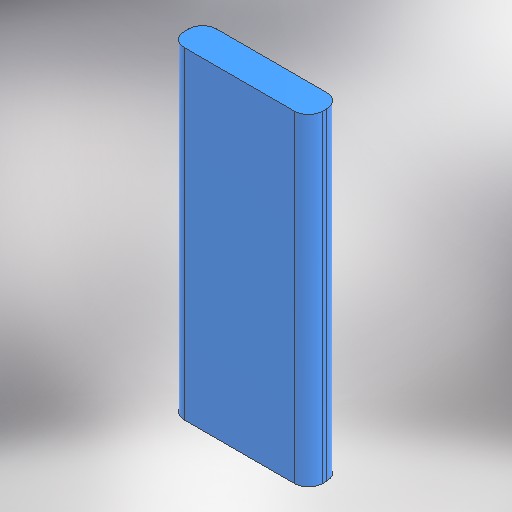
# Autodesk Inventor part: iPod Nano
Saved by Autodesk Inventor 2026.2 (Build 302298000, 298)
## iProperties
Created: 2026-01-13
Part Number: iPod Nano
Material: Generic
Document SubType Name: Modeling
Designer: andyeske
Density: 1 g/cm^3
Appearance: Default
Author: andyeske
Autodesk Inventor part; units mm, degrees
ref_plane "YZ Plane" through (0, 0, 0) normal (1, 0, 0) x (0, 1, 0)
ref_plane "XZ Plane" through (0, 0, 0) normal (0, 1, 0) x (-1, 0, 0)
ref_plane "XY Plane" through (0, 0, 0) normal (0, 0, 1) x (1, 0, 0)
sketch "Sketch1" plane through (0, 0, 0) normal (0, 0, 1) x (1, 0, 0)
  line L0 (-3.81, -8.89) -> (3.81, -8.89)
  line L1 (3.81, -8.89) -> (3.81, 8.89)
  line L2 (3.81, 8.89) -> (-3.81, 8.89)
  line L3 (-3.81, 8.89) -> (-3.81, -8.89)
  line L4 (-3.81, -8.89) -> (3.81, 8.89) construction
  line L5 (3.81, -8.89) -> (-3.81, 8.89) construction
  line L6 (-3.048, 3.048) -> (3.048, 3.048)
  line L7 (3.048, 3.048) -> (3.048, 8.128)
  line L8 (3.048, 8.128) -> (-3.048, 8.128)
  line L9 (-3.048, 8.128) -> (-3.048, 3.048)
  line L10 (-3.048, 3.048) -> (3.048, 8.128) construction
  line L11 (3.048, 3.048) -> (-3.048, 8.128) construction
  circle A0 centre (0, -3.302) radius 2.794
  point P0 (0, 0)
  point P1 (0, 5.588)
  dimension "d0" = 7.62
  dimension "d1" = 17.78
  dimension "d2" = 0.762
  dimension "d3" = 0.762
  dimension "d4" = 0.762
  dimension "d5" = 5.08
  dimension "d6" = 5.588
  dimension "d7" = 5.588
  constraints: 24 end point, 4 midpoint, 4 parallel, 2 horizontal, 2 perpendicular, 1 centre point
  measures "d0" distance of L0.start L0.end
  measures "d1" distance of L2.end L0.start
  measures "d2" distance between parallel lines of L2 L8
  measures "d3" distance between parallel lines of L1 L7
  measures "d4" distance between parallel lines of L3 L9
  measures "d5" distance of L6.end L7.end
  measures "d6" distance from line of A0.centre L0
  measures "d7" diameter of A0
extrude "Extrusion1" add sketch "Sketch1" along normal blind 1.778 contours L3 L2 L1 L0 | L9 L8 L7 L6 | A0
fillet "Fillet1" radius 0.762 4 edges at (3.81, 0, 0) (3.81, 0, 1.778) (-3.81, 0, 1.778) (-3.81, 0, 0)
extrude "Extrusion2" cut sketch "Sketch1" along normal blind 0.0254 contours L9 L8 L7 L6
fillet "Fillet2" radius 0.254 4 edges at (3.048, 8.128, 0.0127) (-3.048, 8.128, 0.0127) (3.048, 3.048, 0.0127) (-3.048, 3.048, 0.0127)
sketch "Sketch2" plane through (0, 0, 0) normal (0, 0, -1) x (-1, 0, 0)
  circle A0 centre (0, -3.302) radius 1.016
  circle A1 centre (0, -3.302) radius 2.794 projected
  point P0 (0, 0)
  dimension "d14" = 2.032
  constraints: 1 centre point, 1 coincident
  measures "d14" diameter of A0
extrude "Extrusion3" add sketch "Sketch2" along normal blind 0.0508
fillet "Fillet3" radius 0.0254 2 edges at (1.016, -3.302, -0.0508) (2.794, -3.302, -0.0508)
sketch "Sketch3" plane through (0, -3.302, -0.0508) normal (0, 0, -1) x (-1, 0, 0)
  line L0 (-0.9463, 2.473) -> (1.05, 2.473) construction
  line L1 (1.05, 2.473) -> (1.05, 1.9797) construction
  line L2 (1.05, 1.9797) -> (-0.9463, 1.9797) construction
  line L3 (-0.9463, 1.9797) -> (-0.9463, 2.473) construction
  line L4 (-2.6797, -0.254) -> (-2.6035, -0.254)
  line L5 (-2.6035, -0.254) -> (-2.6035, 0.254)
  line L6 (-2.6035, 0.254) -> (-2.6797, 0.254)
  line L7 (-2.6797, 0.254) -> (-2.6797, -0.254)
  line L8 (-2.6797, -0.254) -> (-2.6035, 0.254) construction
  line L9 (-2.6035, -0.254) -> (-2.6797, 0.254) construction
  line L10 (0, 0) -> (0, 3.302) construction
  line L11 (-2.5273, 0) -> (-2.2733, 0.254)
  line L12 (-2.2733, 0.254) -> (-2.2733, -0.254)
  line L13 (-2.2733, -0.254) -> (-2.5273, 0)
  line L14 (-2.1971, 0) -> (-1.9431, 0.254)
  line L15 (-1.9431, 0.254) -> (-1.9431, -0.254)
  line L16 (-3.048, 12.192) -> (-3.048, -5.588) projected
  line L17 (-1.9431, -0.254) -> (-2.1971, 0)
  line L18 (2.6797, -0.254) -> (2.6035, -0.254)
  line L19 (2.6035, -0.254) -> (2.6035, 0.254)
  line L20 (2.6035, 0.254) -> (2.6797, 0.254)
  line L21 (2.6797, 0.254) -> (2.6797, -0.254)
  line L22 (2.6797, -0.254) -> (2.6035, 0.254) construction
  line L23 (2.6035, -0.254) -> (2.6797, 0.254) construction
  line L24 (2.5273, 0) -> (2.2733, 0.254)
  line L25 (2.2733, 0.254) -> (2.2733, -0.254)
  line L26 (2.2733, -0.254) -> (2.5273, 0)
  line L27 (2.1971, 0) -> (1.9431, 0.254)
  line L28 (1.9431, 0.254) -> (1.9431, -0.254)
  line L29 (1.9431, -0.254) -> (2.1971, 0)
  line L30 (-0.2936, -2.0988) -> (-0.0396, -2.3528)
  line L31 (-0.0396, -2.3528) -> (-0.2936, -2.6068)
  line L32 (-0.2936, -2.6068) -> (-0.2936, -2.0988)
  line L33 (0.0874, -2.6138) -> (0.1636, -2.6138)
  line L34 (0.1636, -2.6138) -> (0.1636, -2.0919)
  line L35 (0.1636, -2.0919) -> (0.0874, -2.0919)
  line L36 (0.0874, -2.0919) -> (0.0874, -2.6138)
  line L37 (0.0874, -2.6138) -> (0.1636, -2.0919) construction
  line L38 (0.1636, -2.6138) -> (0.0874, -2.0919) construction
  line L39 (0.2398, -2.6138) -> (0.316, -2.6138)
  line L40 (0.316, -2.6138) -> (0.316, -2.0919)
  line L41 (0.316, -2.0919) -> (0.2398, -2.0919)
  line L42 (0.2398, -2.0919) -> (0.2398, -2.6138)
  line L43 (0.2398, -2.6138) -> (0.316, -2.0919) construction
  line L44 (0.316, -2.6138) -> (0.2398, -2.0919) construction
  line L45 (-2.6416, 0) -> (0, 0) construction
  line L46 (-0.903, 2.092) -> (-0.903, 2.473)
  line L47 (-0.903, 2.473) -> (-0.8197, 2.473)
  line L48 (-0.8197, 2.473) -> (-0.7203, 2.2033)
  spline S0 degree 2 poles (-0.7203, 2.2033) (-0.7067, 2.1655) (-0.7003, 2.1469) knots 0 0 0 1 1 1
  spline S1 degree 2 poles (-0.7003, 2.1469) (-0.6933, 2.1675) (-0.6782, 2.2079) knots 0 0 0 1 1 1
  line L49 (-0.6782, 2.2079) -> (-0.5775, 2.473)
  line L50 (-0.5775, 2.473) -> (-0.5031, 2.473)
  line L51 (-0.5031, 2.473) -> (-0.5031, 2.092)
  line L52 (-0.5031, 2.092) -> (-0.5566, 2.092)
  line L53 (-0.5566, 2.092) -> (-0.5566, 2.4109)
  line L54 (-0.5566, 2.4109) -> (-0.6785, 2.092)
  line L55 (-0.6785, 2.092) -> (-0.7285, 2.092)
  line L56 (-0.7285, 2.092) -> (-0.8496, 2.4164)
  line L57 (-0.8496, 2.4164) -> (-0.8496, 2.092)
  line L58 (-0.8496, 2.092) -> (-0.903, 2.092)
  line L59 (-0.4128, 2.092) -> (-0.4128, 2.473)
  line L60 (-0.4128, 2.473) -> (-0.1099, 2.473)
  line L61 (-0.1099, 2.473) -> (-0.1099, 2.428)
  line L62 (-0.1099, 2.428) -> (-0.3573, 2.428)
  line L63 (-0.3573, 2.428) -> (-0.3573, 2.3116)
  line L64 (-0.3573, 2.3116) -> (-0.1256, 2.3116)
  line L65 (-0.1256, 2.3116) -> (-0.1256, 2.2666)
  line L66 (-0.1256, 2.2666) -> (-0.3573, 2.2666)
  line L67 (-0.3573, 2.2666) -> (-0.3573, 2.137)
  line L68 (-0.3573, 2.137) -> (-0.1003, 2.137)
  line L69 (-0.1003, 2.137) -> (-0.1003, 2.092)
  line L70 (-0.1003, 2.092) -> (-0.4128, 2.092)
  line L71 (-0.0246, 2.092) -> (-0.0246, 2.473)
  line L72 (-0.0246, 2.473) -> (0.0324, 2.473)
  line L73 (0.0324, 2.473) -> (0.2522, 2.1739)
  line L74 (0.2522, 2.1739) -> (0.2522, 2.473)
  line L75 (0.2522, 2.473) -> (0.3053, 2.473)
  line L76 (0.3053, 2.473) -> (0.3053, 2.092)
  line L77 (0.3053, 2.092) -> (0.2484, 2.092)
  line L78 (0.2484, 2.092) -> (0.0286, 2.3911)
  line L79 (0.0286, 2.3911) -> (0.0286, 2.092)
  line L80 (0.0286, 2.092) -> (-0.0246, 2.092)
  line L81 (0.673, 2.473) -> (0.7284, 2.473)
  line L82 (0.7284, 2.473) -> (0.7284, 2.2529)
  spline S2 degree 2 poles (0.7284, 2.2529) (0.7284, 2.1954) (0.7, 2.128) (0.6254, 2.0856) (0.5647, 2.0856) knots 0 0 0 1 2 3 3 3
  spline S3 degree 2 poles (0.5647, 2.0856) (0.506, 2.0856) (0.4311, 2.1225) (0.3991, 2.1925) (0.3991, 2.2529) knots 0 0 0 1 2 3 3 3
  line L83 (0.3991, 2.2529) -> (0.3991, 2.473)
  line L84 (0.3991, 2.473) -> (0.4546, 2.473)
  line L85 (0.4546, 2.473) -> (0.4546, 2.2532)
  spline S4 degree 2 poles (0.4546, 2.2532) (0.4546, 2.2038) (0.4749, 2.1568) (0.5243, 2.1312) (0.56, 2.1312) knots 0 0 0 1 2 3 3 3
  spline S5 degree 2 poles (0.56, 2.1312) (0.621, 2.1312) (0.673, 2.1818) (0.673, 2.2532) knots 0 0 0 1 2 2 2
  line L86 (0.673, 2.2532) -> (0.673, 2.473)
  point P0 (2.6416, 0)
  point P1 (0.1255, -2.3528)
  point P2 (0.2779, -2.3528)
  dimension "d18" = 0.254
  dimension "d19" = 0.254
  dimension "d22" = 0.508
  dimension "d23" = 0.254
  dimension "d24" = 3.302
  dimension "d25" = 2.6416
  dimension "d26" = 0.0762
  dimension "d27" = 0.0762
  dimension "d28" = 0.0762
  dimension "d29" = 0.254
  dimension "d30" = 0.508
  dimension "d31" = 0.254
  dimension "d32" = 0.127
  dimension "d33" = 0.0762
  dimension "d34" = 0.0762
  constraints: 82 end point, 11 symmetric about line, 7 parallel, 6 midpoint, 4 equal length, 4 horizontal, 3 perpendicular, 3 point on line, 3 vertical, 1 coincident, 2 other
  measures "d18" distance from line of L11.start L12
  measures "d19" distance from line of L15 L14.start
  measures "d22" distance of L6.end L4.start
  measures "d23" distance from line of L45 L11.end
  measures "d24" distance of L10.start L10.end
  measures "d25" distance of L45.start L10.start
  measures "d26" distance from line of L5 L11.start
  measures "d27" distance from line of L14.start L12
  measures "d28" distance of L5.end L6.end
  measures "d29" distance from line of L45 L14.end
  measures "d30" distance of L31.end L30.start
  measures "d31" horizontal distance of L30.start L30.end
  measures "d32" distance from line of L30.end L36
  measures "d33" distance between parallel lines of L42 L34
  measures "d34" distance of L34.end L35.end
extrude "Extrusion4" cut sketch "Sketch3" against normal blind 0.0127
body "Solid1"
